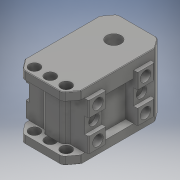
# Autodesk Inventor part: xl320_box
Saved by Autodesk Inventor 2017 (Build 210142000, 142)
## iProperties
Created: 2016-04-25
Part Number: xl320_box
Material: PPS Plastic
Document SubType Name: Modeling
Designer: Ali
Density: 1.637 g/cm^3
Appearance: Smooth - Medium Gray
Author: Ali
Autodesk Inventor part; units mm, degrees
ref_plane "YZ Plane" through (0, 0, 0) normal (1, 0, 0) x (0, 1, 0)
ref_plane "XZ Plane" through (0, 0, 0) normal (0, 1, 0) x (-1, 0, 0)
sketch "Sketch1" plane through (0, 0, 0) normal (0, 0, 1) x (1, 0, 0)
  line L0 (-9.5665, 18.9675) -> (-1.9257, 18.9675)
  line L1 (5.5743, -17.0325) -> (-9.4257, -17.0325)
  line L2 (-102.3302, 36.2807) -> (62.7958, 36.2807) construction
  line L3 (62.7958, 36.2807) -> (62.7958, -27.2193) construction
  line L4 (62.7958, -27.2193) -> (-102.3302, -27.2193) construction
  line L5 (-102.3302, -27.2193) -> (-102.3302, 36.2807) construction
  line L6 (10.0743, -5.0325) -> (8.5743, -5.0325)
  line L7 (10.0743, 12.9675) -> (9.7161, 13.4604)
  line L8 (8.5743, 15.032) -> (5.715, 18.9675)
  line L9 (10.0743, 12.9675) -> (10.0743, 6.9675)
  line L10 (10.0743, -5.0325) -> (10.0743, -11.0325)
  line L11 (-13.9257, -11.0325) -> (-13.9257, -5.0325)
  line L12 (-13.9257, 6.9675) -> (-13.9257, 12.9675)
  line L13 (-13.9257, 12.9675) -> (-13.5676, 13.4604)
  line L14 (-12.4257, 15.032) -> (-9.5665, 18.9675)
  line L15 (-13.9257, -11.0325) -> (-13.5454, -11.5396)
  line L16 (-12.4257, -13.0325) -> (-9.4257, -17.0325)
  line L17 (10.0743, -11.0325) -> (9.694, -11.5396)
  line L18 (8.5743, -13.0325) -> (5.5743, -17.0325)
  line L19 (8.5743, -11.5396) -> (8.5743, -13.0325)
  line L20 (-12.4257, -11.5396) -> (-12.4257, -13.0325)
  line L21 (9.694, -11.5396) -> (8.5743, -11.5396)
  line L22 (-12.4257, -11.5396) -> (-13.5454, -11.5396)
  line L23 (10.0743, 6.9675) -> (8.5743, 6.9675)
  line L24 (-12.4257, 6.9675) -> (-13.9257, 6.9675)
  line L25 (-12.4257, 15.032) -> (-12.4257, 13.4604)
  line L26 (-12.4257, 6.9675) -> (-12.4257, -5.0325)
  line L27 (9.7161, 13.4604) -> (8.5743, 13.4604)
  line L28 (-12.4257, 13.4604) -> (-13.5676, 13.4604)
  line L29 (8.5743, 15.032) -> (8.5743, 13.4604)
  line L30 (8.5743, 6.9675) -> (8.5743, -5.0325)
  circle A0 centre (-7.9257, -14.0325) radius 2
  circle A1 centre (-1.9257, -14.0325) radius 2
  circle A2 centre (4.0743, -14.0325) radius 2
  line L31 (-12.4257, -5.0325) -> (-13.9257, -5.0325)
  line L32 (-16.1935, 9.9675) -> (-1.9257, 9.9675) construction
  line L33 (-19.3681, -14.0325) -> (14.6602, -14.0325) construction
  line L34 (-12.4257, -11.5396) -> (-1.9257, -11.5396) construction
  line L35 (-1.9257, -11.5396) -> (-1.9257, 18.9675) construction
  line L36 (-1.9257, -11.5396) -> (8.5743, -11.5396) construction
  line L37 (-1.9257, 18.9675) -> (5.715, 18.9675)
  line L38 (-1.9257, 9.9675) -> (12.3065, 9.9675) construction
  point P0 (0, 0)
  point P1 (-13.9257, 18.9675)
  point P2 (10.0743, -17.0325)
  point P3 (10.0743, 18.9675)
  point P4 (-13.9257, -17.0325)
  dimension "d0" = 36
  dimension "d1" = 24
  dimension "d15" = 6
  dimension "d17" = 6
  dimension "d48" = 4
  dimension "d49" = 3
  dimension "d50" = 4
  dimension "d51" = 4
  dimension "d52" = 12
  dimension "d53" = 6
  dimension "d102" = 25
  dimension "d103" = 12
  dimension "d104" = 21
  dimension "d107" = 15
  dimension "d109" = 9
  dimension "d110" = 24
  dimension "d111" = 12
  dimension "d123" = 36
  dimension "d127" = 36
  constraints: 70 end point, 16 collinear, 16 perpendicular, 13 point on line, 7 horizontal, 7 vertical, 6 parallel, 4 equal length, 3 centre point, 2 other
  measures "d0" distance of point (10.074, 18.967) point (10.074, -17.033)
  measures "d1" distance of point (-13.926, 18.967) point (10.074, 18.967)
  measures "d15" distance of L7.start point (10.074, 18.967)
  measures "d17" distance of L12.end point (-13.926, 18.967)
  measures "d48" diameter of A0
  measures "d49" distance from line of L1 A0.centre
  measures "d50" diameter of A1
  measures "d51" diameter of A2
  measures "d52" distance of A2.centre A0.centre
  measures "d53" distance of A2.centre A1.centre
  measures "d102" distance between parallel lines of L22 L28
  measures "d103" distance between parallel lines of L6 L23
  measures "d104" distance between parallel lines of L30 L26
  measures "d107" distance of L1.start L1.end
  measures "d109" distance between parallel lines of L0 L32
  measures "d110" distance between parallel lines of L33 L32
  measures "d111" distance between parallel lines of L1 L6
  measures "d123" angle of L8 L35
  measures "d127" distance between parallel lines of L1 L37
extrude "Extrusion1" add sketch "Sketch1" along normal blind 24
sketch "Sketch2" plane through (10.0743, -11.0325, 0) normal (1, 0, 0) x (0, 0, -1)
  line L0 (-156.4574, 52.5662) -> (8.6686, 52.5662) construction
  line L1 (8.6686, 52.5662) -> (8.6686, -10.9338) construction
  line L2 (8.6686, -10.9338) -> (-156.4574, -10.9338) construction
  line L3 (-156.4574, -10.9338) -> (-156.4574, 52.5662) construction
  line L4 (0, 24.493) -> (0, 24) projected
  line L5 (-24, 24) -> (-24, 24.493) projected
  line L6 (0, 24) -> (-24, 24) projected
  line L7 (0, 0) -> (0, -0.507) projected
  line L8 (0, 0) -> (-24, 0) projected
  line L9 (-24, -0.507) -> (-24, 0) projected
  line L10 (0, -6) -> (-24, -6) projected
  line L11 (-21, -6) -> (-3, -6)
  line L12 (-3, -6) -> (-3, -0.507)
  line L13 (-3, -0.507) -> (-21, -0.507)
  line L14 (-21, -0.507) -> (-21, -6)
  line L15 (0, -0.507) -> (-24, -0.507) projected
  line L16 (0, 24.493) -> (-24, 24.493) projected
  point P0 (0, 11.0325)
  dimension "d28" = 3
  dimension "d29" = 3
  constraints: 8 end point, 2 parallel, 1 collinear, 1 horizontal, 1 perpendicular, 1 point on line, 2 other
  measures "d28" distance between parallel lines of L9 L14
  measures "d29" distance between parallel lines of L7 L12
extrude "Extrusion2" cut sketch "Sketch2" against normal through all contours L12 L10 L14 L13
sketch "Sketch3" plane through (-9.5665, 18.9675, 0) normal (0, 1, 0) x (1, 0, 0)
  line L0 (-2.8593, -3.255) -> (-8.7726, -3.255)
  line L1 (-8.7726, -3.255) -> (-8.7726, 0)
  line L2 (-8.7726, 0) -> (-2.8593, 0)
  line L3 (-2.8593, -20.745) -> (-8.7726, -20.745)
  line L4 (-8.7726, -20.745) -> (-8.7726, -24)
  line L5 (-8.7726, -24) -> (-2.8593, -24)
  line L6 (-8.7726, -15) -> (-2.8593, -15)
  line L7 (-2.8593, -9) -> (-8.7726, -9)
  line L8 (-8.7726, -9) -> (-8.7726, -15)
  line L9 (0, 0) -> (0, -24) projected
  line L10 (15.2815, 0) -> (15.2815, -24) projected
  line L11 (0, -12) -> (15.2815, -12)
  line L12 (7.6407, -12) -> (7.6407, -7.4528)
  line L13 (-2.8593, 0) -> (-2.8593, -24) projected
  line L14 (18.1407, -3.255) -> (24.0541, -3.255)
  line L15 (24.0541, -3.255) -> (24.0541, 0)
  line L16 (24.0541, 0) -> (18.1407, 0)
  line L17 (18.1407, -20.745) -> (24.0541, -20.745)
  line L18 (24.0541, -20.745) -> (24.0541, -24)
  line L19 (24.0541, -24) -> (18.1407, -24)
  line L20 (24.0541, -15) -> (18.1407, -15)
  line L21 (18.1407, -9) -> (24.0541, -9)
  line L22 (24.0541, -9) -> (24.0541, -15)
  line L23 (18.1407, 0) -> (18.1407, -24)
  point P0 (-8.7726, -12)
  point P1 (24.0541, -12)
  dimension "d88" = 6
  constraints: 42 end point, 15 symmetric about line, 14 point on line, 4 midpoint, 2 horizontal, 2 parallel, 1 perpendicular, 1 vertical
  measures "d88" distance between parallel lines of L7 L6
extrude "Extrusion3" cut sketch "Sketch3" against normal through all
sketch "Sketch4" plane through (8.5743, -13.0325, 0) normal (1, 0, 0) x (0, 0, -1)
  line L0 (-15, 8) -> (-20.745, 8) projected
  line L1 (-20.745, 8) -> (-3.255, 8)
  line L2 (-3.255, 8) -> (-3.255, 20)
  line L3 (-3.255, 20) -> (-20.745, 20)
  line L4 (-20.745, 20) -> (-20.745, 8)
  constraints: 8 end point, 2 parallel, 1 horizontal, 1 perpendicular
extrude "Extrusion4" cut sketch "Sketch4" against normal blind 3
sketch "Sketch5" plane through (-12.4257, -13.0325, 0) normal (-1, 0, 0) x (0, 0, 1)
  line L0 (9, 8) -> (9, 1.493) projected
  line L1 (15, 26.493) -> (20.745, 26.493) projected
  line L2 (20.745, 26.493) -> (20.745, 20) projected
  line L3 (15, 20) -> (20.745, 20) projected
  line L4 (15, 26.493) -> (15, 20) projected
  line L5 (9, 26.493) -> (9, 20) projected
  line L6 (3.255, 20) -> (9, 20) projected
  line L7 (3.255, 26.493) -> (3.255, 20) projected
  line L8 (3.255, 26.493) -> (9, 26.493) projected
  line L9 (0, 0) -> (0, 28.0646) projected
  line L10 (0, 0) -> (3, 0) projected
  line L11 (3, 0) -> (3, 1.493) projected
  line L12 (3.255, 1.493) -> (3, 1.493) projected
  line L13 (3.255, 8) -> (3.255, 1.493) projected
  line L14 (3.255, 8) -> (9, 8) projected
  line L15 (9, 8) -> (9, 1.493) projected
  line L16 (15, 1.493) -> (9, 1.493) projected
  line L17 (15, 8) -> (15, 1.493) projected
  line L18 (15, 8) -> (20.745, 8) projected
  line L19 (20.745, 8) -> (20.745, 1.493) projected
  line L20 (21, 1.493) -> (20.745, 1.493) projected
  line L21 (21, 1.493) -> (21, 0) projected
  line L22 (21, 0) -> (24, 0) projected
  line L23 (24, 28.0646) -> (24, 0) projected
  line L24 (0, 28.0646) -> (24, 28.0646) projected
  line L25 (3.255, 8) -> (9, 8) projected
  line L26 (15, 20) -> (20.745, 20) projected
  line L27 (3.255, 8) -> (20.745, 8)
  line L28 (20.745, 8) -> (20.745, 20)
  line L29 (20.745, 20) -> (3.255, 20)
  line L30 (3.255, 20) -> (3.255, 8)
  constraints: 8 end point, 2 parallel, 1 horizontal, 1 perpendicular
extrude "Extrusion5" cut sketch "Sketch5" against normal blind 3 contours L14 L30 L6 L29 L3 L28 L18 L27
sketch "Sketch6" plane through (0, 0, 24) normal (0, 0, 1) x (1, 0, 0)
  circle A0 centre (-7.9257, -14.0325) radius 2 projected
  circle A1 centre (-1.9257, 9.9675) radius 2.75
  line L0 (-9.5665, 18.9675) -> (5.715, 18.9675) projected
  line L1 (-1.9257, 18.9675) -> (-1.9257, -17.0325) construction
  line L2 (5.5743, -17.0325) -> (-9.4257, -17.0325) projected
  circle A2 centre (-1.9257, 9.9675) radius 8.8 construction
  point P0 (0, 0)
  dimension "d59" = 24
  dimension "d60" = 17.6
  dimension "d97" = 5.5
  constraints: 2 centre point, 2 end point, 2 midpoint, 1 coincident, 1 point on line
  measures "d59" vertical distance of A1.centre A0.centre
  measures "d60" diameter of A2
  measures "d97" diameter of A1
extrude "Extrusion6" cut sketch "Sketch6" against normal blind 5 contours A1
sketch "Sketch7" plane through (0, 0, 0) normal (0, 0, -1) x (-1, 0, 0)
  circle A0 centre (-4.0743, -14.0325) radius 2 projected
  circle A1 centre (1.9257, -14.0325) radius 2 projected
  circle A2 centre (7.9257, -14.0325) radius 2 projected
  circle A3 centre (-4.0743, 9.9675) radius 2
  circle A4 centre (1.9257, 9.9675) radius 2
  circle A5 centre (7.9257, 9.9675) radius 2
  line L0 (-4.0743, -14.0325) -> (-4.0743, 17.2425) construction
  line L1 (1.9257, -14.0325) -> (1.9257, 17.2425) construction
  line L2 (7.9257, -14.0325) -> (7.9257, 17.2425) construction
  line L3 (-14.7465, 9.9675) -> (18.051, 9.9675) construction
  point P0 (0, 0)
  dimension "d63" = 4
  dimension "d64" = 4
  dimension "d65" = 4
  dimension "d66" = 24
  constraints: 8 end point, 6 point on line, 3 centre point, 3 vertical, 1 horizontal
  measures "d63" diameter of A3
  measures "d64" diameter of A4
  measures "d65" diameter of A5
  measures "d66" distance from line of L0.start L3
extrude "Extrusion7" cut sketch "Sketch7" against normal blind 3 contours A3 | A4 | A5
sketch "Sketch8" plane through (10.0743, 6.9682, 3.255) normal (1, 0, 0) x (0, 0, -1)
  line L0 (-17.49, 5.9993) -> (-17.49, -0.0007) projected
  line L1 (-11.745, -0.0007) -> (-17.49, -0.0007) projected
  line L2 (-11.745, -0.0007) -> (-11.745, 5.9993) projected
  line L3 (-11.745, 5.9993) -> (-17.49, 5.9993) projected
  line L4 (0, -0.0007) -> (0, 5.9993) projected
  line L5 (0, 5.9993) -> (-5.745, 5.9993) projected
  line L6 (-5.745, 5.9993) -> (-5.745, -0.0007) projected
  line L7 (0, -0.0007) -> (-5.745, -0.0007) projected
  line L8 (0, -18.0007) -> (0, -12.0007) projected
  line L9 (0, -12.0007) -> (-5.745, -12.0007) projected
  line L10 (-5.745, -12.0007) -> (-5.745, -18.0007) projected
  line L11 (0, -18.0007) -> (-5.745, -18.0007) projected
  line L12 (-17.49, -12.0007) -> (-17.49, -18.0007) projected
  line L13 (-11.745, -18.0007) -> (-17.49, -18.0007) projected
  line L14 (-11.745, -18.0007) -> (-11.745, -12.0007) projected
  line L15 (-11.745, -12.0007) -> (-17.49, -12.0007) projected
  line L16 (-20.745, -20.0007) -> (-20.745, 8.0638) projected
  line L17 (3.255, 8.0638) -> (3.255, -20.0007) projected
  circle A0 centre (-14.745, 2.9993) radius 2
  line L18 (3.255, 11.9993) -> (-20.745, 11.9993) projected
  circle A1 centre (-8.745, 2.9993) radius 2
  circle A2 centre (-2.745, 2.9993) radius 2
  circle A3 centre (-14.745, -15.0007) radius 2
  circle A4 centre (-8.745, -15.0007) radius 2
  circle A5 centre (-2.745, -15.0007) radius 2
  dimension "d133" = 4
  dimension "d134" = 6
  dimension "d135" = 18
  dimension "d136" = 9
  dimension "d139" = 6
  dimension "d142" = 18
  constraints: 6 centre point, 1 horizontal, 1 vertical, 10 other
  measures "d133" diameter of A0
  measures "d134" distance from line of L16 A0.centre
  measures "d135" distance from line of L17 A0.centre
  measures "d136" distance from line of L18 A0.centre
  measures "d139" distance of A0.centre A1.centre
  measures "d142" distance of A0.centre A3.centre
extrude "Extrusion8" cut sketch "Sketch8" against normal blind 3 contours A0 | A1 | A2 | A3 | A4 | A5
ref_plane "Work Plane1" through (-1.9257, -13.0325, 0) normal (1, 0, 0) x (0, 0, -1)
mirror "Mirror1" about plane through (-1.9257, -13.0325, 0) normal (1, 0, 0) of "Extrusion8"
sketch "Sketch9" plane through (5.5743, -13.0325, 0) normal (1, 0, 0) x (0, 0, -1)
  line L0 (-17.245, 20.534) -> (-17.245, 8)
  line L1 (-17.245, 20.534) -> (-20.745, 20.534)
  line L2 (-3.255, 8) -> (-20.745, 8) projected
  line L3 (-3.255, 20) -> (-3.255, 8) projected
  line L4 (-20.745, 20) -> (-3.255, 20) projected
  line L5 (-20.745, 8) -> (-20.745, 20) projected
  line L6 (-20.745, 20) -> (-3.255, 20) projected
  line L7 (-20.745, 8) -> (-20.745, 1.493) projected
  line L8 (-17.245, 20) -> (-20.745, 20)
  line L9 (-20.745, 20) -> (-20.745, 8)
  line L10 (-20.745, 8) -> (-17.245, 8)
  line L11 (-17.245, 8) -> (-17.245, 20)
  point P0 (-3.255, 8.534)
  point P1 (0, 13.0325)
  dimension "d132" = 3.5
  constraints: 12 end point, 3 point on line, 2 horizontal, 2 parallel, 1 perpendicular
  measures "d132" distance between parallel lines of L0 L5
extrude "Extrusion9" add sketch "Sketch9" along normal up to surface (3 mm away) contours L0 L2 L5 L4
mirror "Mirror2" about plane through (-1.9257, -13.0325, 0) normal (1, 0, 0) of "Extrusion9"
chamfer "Chamfer2" distance 0.8 angle 45 2 edges at (-12.4257, 0.9675, 17.245) (8.5743, 0.9675, 17.245)
fillet "Fillet1" radius 2 6 edges at (-9.5665, 18.9675, 12) (5.715, 18.9675, 12) (-9.4257, -17.0325, 22.5) (-9.4257, -17.0325, 1.5) (5.5743, -17.0325, 22.5) (5.5743, -17.0325, 1.5)
sketch "Sketch10" plane through (-12.4257, -11.5396, 3) normal (0, -1, 0) x (1, 0, 0)
  line L0 (21, 0) -> (0, 0) projected
  line L1 (4, 18) -> (17, 18) projected
  line L2 (14.25, 0) -> (6.75, 0)
  line L3 (6.75, 0) -> (6.75, 18)
  line L4 (6.75, 18) -> (14.25, 18)
  line L5 (14.25, 18) -> (14.25, 0)
  line L6 (10.5, -3.8604) -> (10.5, 22.9969) construction
  line L7 (17, 0) -> (4, 0) projected
  point P0 (12.4257, -3)
  point P1 (10.5, 0)
  point P2 (10.5, 0)
  dimension "d93" = 7.5
  constraints: 10 end point, 4 point on line, 2 midpoint, 2 parallel, 1 horizontal, 1 perpendicular, 1 vertical
  measures "d93" distance between parallel lines of L3 L5
extrude "Extrusion10" add sketch "Sketch10" along normal blind 1.5
fillet "Fillet2" radius 1.5 4 edges at (1.8243, -11.5396, 12) (-5.6757, -11.5396, 12) (1.8243, -13.0396, 12) (-5.6757, -13.0396, 12)
chamfer "Chamfer3" distance 0.2 angle 45 45 edges at (-1.9257, 18.9675, 0) (-9.4554, 18.7495, 0) (-11.2956, 16.5875, 0) (5.604, 18.7495, 0) (7.4442, 16.5875, 0) (-12.4257, 0.9998, 0) (-9.4554, 18.7495, 24) (-1.9257, 18.9675, 24) (5.604, 18.7495, 24) (7.4442, 16.5875, 24) (-11.2956, 16.5875, 24) (-12.4257, 0.9998, 24) (8.5743, 0.9998, 24) (-1.9257, -17.0325, 24) (5.4687, -16.8214, 24) (7.3743, -14.6325, 24) (-9.3201, -16.8214, 24) (-11.2257, -14.6325, 24) (-11.2257, -14.6325, 0) (-9.3201, -16.8214, 0) (-1.9257, -17.0325, 0) (5.4687, -16.8214, 0) (7.3743, -14.6325, 0) (-12.4257, 15.032, 12) (8.5743, 15.032, 12) (8.5743, -13.0325, 22.5) (8.5743, -13.0325, 1.5) (-12.4257, -13.0325, 22.5) (-12.4257, -13.0325, 1.5) (-13.9257, 9.9675, 20.745) (-13.9257, 9.9675, 15) (-13.9257, -8.0325, 20.745) (-13.9257, -8.0325, 15) (-13.9257, -8.0325, 9) (-13.9257, -8.0325, 3.255) (-13.9257, 9.9675, 3.255) (-13.9257, 9.9675, 9) (-13.9257, 6.9675, 6.1275) (-13.9257, 6.9675, 17.8725) (-13.9257, -5.0325, 17.8725) (-13.9257, -5.0325, 6.1275) (10.0743, 6.9675, 17.8725) (10.0743, 6.9675, 6.1275) (10.0743, -5.0325, 6.1275) (10.0743, -5.0325, 17.8725)
equation "\"d17\" = d15"
body "Solid1"
